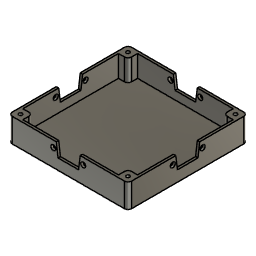
TRARM02_Base_Bottom_100x100x20 (Autodesk Fusion 360 design; units mm, degrees)
Autodesk Fusion 360 part; units mm, degrees
sketch "스케치1" plane through (0, 0, 0) normal (0, 0, 1) x (1, 0, 0)
  line L0 (0, 0) -> (100, 0)
  line L1 (100, 0) -> (100, 100)
  line L2 (100, 100) -> (0, 100)
  line L3 (0, 100) -> (0, 0)
  dimension "d25" = 100
  dimension "d26" = 100
  constraint horizontal L0
  constraint vertical L1
  constraint horizontal L2
  constraint vertical L3
  constraint coincident L0.start L3.end
  measures "d25" distance of L0.start L0.end
  measures "d26" distance of L0.start L2.end
extrude "돌출4" add sketch "스케치1" along normal blind 2
sketch "스케치7" plane through (0, 0, 2) normal (0, 0, 1) x (-1, 0, 0)
  line L0 (0, -100) -> (-100, -100)
  line L1 (-100, -100) -> (-100, 0)
  line L2 (-100, 0) -> (0, 0)
  line L3 (0, 0) -> (0, -100)
  line L4 (-10, -98) -> (-90, -98)
  line L5 (-98, -90) -> (-98, -10)
  line L6 (-90, -2) -> (-10, -2)
  line L7 (-2, -10) -> (-2, -90)
  line L8 (-2, -90) -> (-10, -90)
  line L9 (-10, -90) -> (-10, -98)
  line L10 (-90, -98) -> (-90, -90)
  line L11 (-90, -90) -> (-98, -90)
  line L12 (-2, -10) -> (-10, -10)
  line L13 (-10, -10) -> (-10, -2)
  line L14 (-90, -2) -> (-90, -10)
  line L15 (-90, -10) -> (-98, -10)
  point P0 (0, -100)
  point P1 (-100, 0)
  dimension "d46" = 2
  dimension "d47" = 2
  dimension "d49" = 2
  dimension "d50" = 2
  dimension "d85" = 10
  dimension "d86" = 10
  dimension "d91" = 10
  dimension "d92" = 10
  constraint horizontal L0
  constraint vertical L1
  constraint horizontal L2
  constraint vertical L3
  constraint coincident P1 L1.end
  constraint coincident P0 L0.start
  constraint horizontal L4
  constraint vertical L5
  constraint horizontal L6
  constraint vertical L7
  constraint perpendicular L7 L8
  constraint perpendicular L4 L9
  constraint perpendicular L4 L10
  constraint perpendicular L5 L11
  constraint perpendicular L7 L12
  constraint perpendicular L6 L13
  constraint perpendicular L6 L14
  constraint perpendicular L5 L15
  constraint equal L9 L10
  constraint equal L8 L11
  constraint equal L13 L14
  constraint equal L12 L15
  measures "d46" distance of L3 L7
  measures "d47" distance of L0 L4
  measures "d49" distance of L1 L5
  measures "d50" distance of L2 L6
  measures "d85" distance of P0 L9
  measures "d86" distance of P0 L8
  measures "d91" distance of P1 L14
  measures "d92" distance of P1 L15
extrude "돌출7" add sketch "스케치7" along normal blind 18
fillet "모깎기1" radius 3 4 edges at (100, 0, 10) (0, 0, 10) (100, 100, 10) (0, 100, 10)
fillet "모깎기1" radius 3 4 edges at (10, 90, 11) (10, 10, 11) (90, 10, 11) (90, 90, 11)
sketch "스케치9" plane through (0, 0, 0) normal (0, -1, 0) x (1, 0, 0)
  line L0 (41.4, 9) -> (40, 20)
  line L1 (90, 20) -> (10, 20)
  line L2 (41.4, 9) -> (58.6, 9)
  line L3 (58.6, 9) -> (60, 20)
  line L4 (40, 20) -> (60, 20)
  circle A0 centre (62.5, 14.5) radius 2.1
  circle A1 centre (37.5, 14.5) radius 2.1
  point P0 (50, 20)
  point P1 (10, 20)
  point P2 (90, 20)
  dimension "d72" = 17.2
  dimension "d73" = 50
  dimension "d74" = 20
  dimension "d75" = 11
  dimension "d76" = 4.2
  dimension "d77" = 4.2
  dimension "d78" = 25
  dimension "d81" = 5.5
  dimension "d82" = 12.5
  constraint coincident L1 P0
  constraint coincident L3.end L1
  constraint coincident L1 L0.end
  constraint midpoint P0 L4
  constraint equal L0 L3
  constraint horizontal A0.centre A1.centre
  measures "d72" distance of L0.start L2.end
  measures "d73" horizontal distance of origin P0
  measures "d74" distance of L3.end L0.end
  measures "d75" distance of L2 L4
  measures "d76" diameter of A0
  measures "d77" diameter of A1
  measures "d78" distance of A0.centre A1.centre
  measures "d81" distance of L2 A1.centre
  measures "d82" horizontal distance of P0 A1.centre
extrude "돌출9" cut sketch "스케치9" against normal blind 100
sketch "스케치11" plane through (0, 0, 20) normal (0, 0, 1) x (-1, 0, 0)
  circle A0 centre (-5, -95) radius 1.45
  circle A1 centre (-95, -95) radius 1.45
  circle A2 centre (-95, -5) radius 1.45
  circle A3 centre (-5, -5) radius 1.45
  line L0 (0, -97) -> (0, -3)
  line L1 (-3, 0) -> (-40, 0)
  line L2 (-60, 0) -> (-97, 0)
  line L3 (-100, -3) -> (-100, -97)
  line L4 (-97, -100) -> (-60, -100)
  line L5 (-40, -100) -> (-3, -100)
  line L6 (-97, -100) -> (-60, -100)
  dimension "d93" = 2.9
  dimension "d103" = 5
  dimension "d108" = 2.9
  dimension "d109" = 90
  dimension "d110" = 90
  constraint horizontal A0.centre A1.centre
  constraint equal A2 A3
  constraint vertical A0.centre A3.centre
  constraint horizontal A2.centre A3.centre
  constraint vertical A1.centre A2.centre
  constraint equal A0 A1
  measures "d93" diameter of A3
  measures "d103" distance of A0.centre L0
  measures "d108" diameter of A0
  measures "d109" distance of A0.centre A1.centre
  measures "d110" distance of A0.centre A3.centre
extrude "돌출10" cut sketch "스케치11" against normal blind 20
sketch "스케치12" plane through (0, 0, 0) normal (-1, 0, 0) x (0, -1, 0)
  line L0 (-58.6, 9) -> (-41.4, 9)
  circle A0 centre (-62.5, 14.5) radius 2.1
  line L1 (-58.6, 9) -> (-60, 20)
  line L2 (-60, 20) -> (-40, 20)
  line L3 (-41.4, 9) -> (-40, 20)
  circle A1 centre (-37.5, 14.5) radius 2.1
  line L4 (-97, 20) -> (-3, 20)
  point P0 (-64, 20)
  point P1 (-100, 0)
  point P2 (-50, 20)
  point P3 (-90, 20)
  dimension "d115" = 17.2
  dimension "d117" = 20
  dimension "d118" = 11
  dimension "d119" = 4.2
  dimension "d120" = 4.2
  dimension "d121" = 25
  dimension "d122" = 5.5
  dimension "d123" = 12.5
  dimension "d124" = 50
  constraint midpoint P2 L2
  constraint equal L1 L3
  constraint horizontal A1.centre A0.centre
  constraint parallel L2 L4
  constraint coincident P2 L4
  measures "d115" distance of L0.start L0.end
  measures "d117" distance of L2.end L1.end
  measures "d118" distance of L0 L2
  measures "d119" diameter of A1
  measures "d120" diameter of A0
  measures "d121" distance of A1.centre A0.centre
  measures "d122" distance of A0.centre L0
  measures "d123" horizontal distance of A0.centre P2
  measures "d124" horizontal distance of origin P2
extrude "돌출11" cut sketch "스케치12" against normal blind 100
